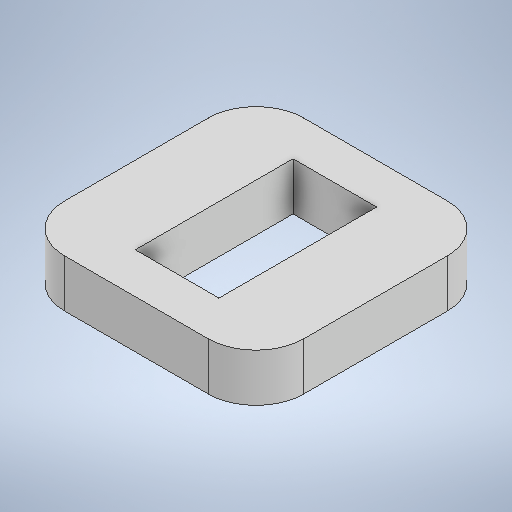
# Autodesk Inventor part: Test_TOF_hole
Saved by Autodesk Inventor 2025 (Build 290162000, 162)
## iProperties
Created: 2026-03-10
Part Number: Test_TOF_hole
Material: Générique
Document SubType Name: Modeling
Designer: luc4s
Density: 1 g/cm^3
Appearance: Par défaut
Author: luc4s
## iProperties of the stored document Test_TOF_hole_Impression 3D.ipt
Created: 2026-03-10
Part Number: Test_TOF_hole_Impression 3D
Material: Générique
Document SubType Name: Modeling
Designer: luc4s
Density: 1 g/cm^3
Appearance: Par défaut
Author: luc4s
Autodesk Inventor part; units mm, degrees
ref_plane "YZ Plane" through (0, 0, 0) normal (1, 0, 0) x (0, 1, 0)
ref_plane "XZ Plane" through (0, 0, 0) normal (0, 1, 0) x (-1, 0, 0)
ref_plane "XY Plane" through (0, 0, 0) normal (0, 0, 1) x (1, 0, 0)
sketch "Esquisse1" plane through (0, 0, 0) normal (0, 1, 0) x (-1, 0, 0)
  line L0 (5, 5) -> (-5, 5)
  line L1 (-5, 5) -> (-5, -5)
  line L2 (-5, -5) -> (5, -5)
  line L3 (5, -5) -> (5, 5)
  line L4 (5, 5) -> (-5, -5) construction
  line L5 (5, -5) -> (-5, 5) construction
  line L6 (-1.75, -3.3) -> (1.75, -3.3)
  line L7 (1.75, -3.3) -> (1.75, 3.3)
  line L8 (1.75, 3.3) -> (-1.75, 3.3)
  line L9 (-1.75, 3.3) -> (-1.75, -3.3)
  line L10 (-1.75, -3.3) -> (1.75, 3.3) construction
  line L11 (1.75, -3.3) -> (-1.75, 3.3) construction
  point P0 (0, 0)
  point P1 (0, 0)
  point P2 (15, 0)
  point P3 (0, 0)
  point P4 (0, 0)
  dimension "d0" = 10
  dimension "d1" = 10
  dimension "d2" = 6.6
  dimension "d3" = 3.5
  dimension "d4" = 15
  dimension "d5" = 5
  dimension "d6" = 5
  constraints: 24 end point, 4 parallel, 3 midpoint, 3 perpendicular, 2 horizontal, 1 coincident
  measures "d0" distance of L2.end L0.start
  measures "d1" distance of L1.end L2.end
  measures "d2" distance of L8.end L6.start
  measures "d3" distance of L7.end L8.end
  measures "d4" distance of point (15, 0) point (0, 0)
  measures "d5" distance from line of L2 point (0, 0)
  measures "d6" distance from line of L1 point (0, 0)
extrude "Extrusion1" add sketch "Esquisse1" along normal blind 2
fillet "Congé1" radius 2 4 edges at (5, 1, 5) (-5, 1, 5) (-5, 1, -5) (5, 1, -5)
